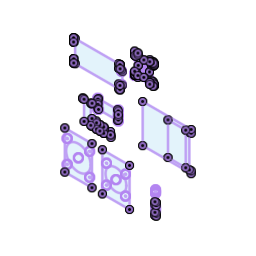
panels (Autodesk Fusion 360 design; units mm, degrees)
Autodesk Fusion 360 part; units mm, degrees
(part 1 of 2)
sketch "back construction" plane through (0, 0, 0) normal (0, 1, 0) x (1, 0, 0)
  line L0 (63.5, -61) -> (184.5, -61) construction
  line L1 (184.5, -61) -> (184.5, -120.5) construction
  line L2 (184.5, -120.5) -> (63.5, -120.5) construction
  line L3 (63.5, -120.5) -> (63.5, -61) construction
  line L4 (31.5, -5) -> (140.5, -5) construction
  line L5 (140.5, -5) -> (140.5, 39.5) construction
  line L6 (140.5, 39.5) -> (31.5, 39.5) construction
  line L7 (31.5, 39.5) -> (31.5, -5) construction
  line L8 (28.5, 32) -> (-8.5, 32)
  line L9 (-8.5, 32) -> (-8.5, -74)
  line L10 (-8.5, -74) -> (28.5, -74)
  line L11 (28.5, -74) -> (28.5, 32)
  line L12 (-15.5, -74) -> (35.5, -74)
  line L13 (35.5, -74) -> (35.5, -77)
  line L14 (35.5, -77) -> (-15.5, -77)
  line L15 (-15.5, -77) -> (-15.5, -74)
  line L16 (35, 34.5) -> (59, 34.5)
  line L17 (59, 34.5) -> (59, -3.5)
  line L18 (59, -3.5) -> (35, -3.5)
  line L19 (35, -3.5) -> (35, 34.5)
  line L20 (60.5, 34.5) -> (78.5, 34.5)
  line L21 (78.5, 34.5) -> (78.5, 4.5)
  line L22 (78.5, 4.5) -> (60.5, 4.5)
  line L23 (60.5, 4.5) -> (60.5, 34.5)
  line L24 (100, 34.5) -> (100, 4.5)
  line L25 (100, 4.5) -> (82, 4.5)
  line L26 (82, 4.5) -> (82, 34.5)
  line L27 (82, 34.5) -> (100, 34.5)
  line L28 (102, 34.5) -> (140, 34.5)
  line L29 (140, 34.5) -> (140, 23.5)
  line L30 (140, 23.5) -> (102, 23.5)
  line L31 (102, 23.5) -> (102, 34.5)
  line L32 (104.5, 23.5) -> (137.5, 23.5)
  line L33 (137.5, 23.5) -> (137.5, 7.5)
  line L34 (137.5, 7.5) -> (104.5, 7.5)
  line L35 (104.5, 7.5) -> (104.5, 23.5)
  circle A0 centre (180.5, -116.5) radius 4 construction
  circle A1 centre (180.5, -91) radius 4 construction
  circle A2 centre (180.5, -65) radius 4 construction
  circle A3 centre (67.5, -116.5) radius 4 construction
  circle A4 centre (67.5, -91) radius 4 construction
  circle A5 centre (67.5, -65) radius 4 construction
  line L36 (180.5, -116.5) -> (67.5, -116.5) construction
  line L37 (67.5, -116.5) -> (67.5, -65) construction
  line L38 (67.5, -65) -> (180.5, -65) construction
  line L39 (180.5, -65) -> (180.5, -116.5) construction
  line L40 (180.5, -95) -> (180.5, -112.5)
  line L41 (176.5, -116.5) -> (71.5, -116.5)
  line L42 (67.5, -112.5) -> (67.5, -95)
  line L43 (67.5, -87) -> (67.5, -69)
  line L44 (71.5, -65) -> (176.5, -65)
  line L45 (180.5, -69) -> (180.5, -87)
  arc A6 (180.5, -69) -> (176.5, -65) centre (180.5, -65) ccw
  line L46 (180.5, -65) -> (180.5, -69) construction
  line L47 (180.5, -65) -> (176.5, -65) construction
  arc A7 (176.5, -116.5) -> (180.5, -112.5) centre (180.5, -116.5) ccw
  line L48 (180.5, -116.5) -> (176.5, -116.5) construction
  line L49 (180.5, -116.5) -> (180.5, -112.5) construction
  arc A8 (67.5, -112.5) -> (71.5, -116.5) centre (67.5, -116.5) ccw
  line L50 (67.5, -116.5) -> (67.5, -112.5) construction
  line L51 (67.5, -116.5) -> (71.5, -116.5) construction
  arc A9 (67.5, -87) -> (67.5, -95) centre (67.5, -91) ccw
  line L52 (67.5, -91) -> (67.5, -87) construction
  line L53 (67.5, -91) -> (67.5, -95) construction
  arc A10 (71.5, -65) -> (67.5, -69) centre (67.5, -65) ccw
  line L54 (67.5, -65) -> (71.5, -65) construction
  line L55 (67.5, -65) -> (67.5, -69) construction
  arc A11 (180.5, -95) -> (180.5, -87) centre (180.5, -91) ccw
  line L56 (180.5, -91) -> (180.5, -95) construction
  line L57 (180.5, -91) -> (180.5, -87) construction
  line L58 (240.5, -148.5) -> (-54.5, -148.5)
  line L59 (-54.5, -148.5) -> (-54.5, 62.5)
  line L60 (-54.5, 62.5) -> (240.5, 62.5)
  line L61 (240.5, 62.5) -> (240.5, -148.5)
  dimension "d10" = 121
  dimension "d11" = 59.5
  dimension "d12" = 109
  dimension "d13" = 44.5
  dimension "d14" = 37
  dimension "d15" = 106
  dimension "d16" = 51
  dimension "d17" = 3
  dimension "d18" = 3
  dimension "d19" = 7
  dimension "d20" = 35
  dimension "d21" = 56
  dimension "d22" = 7.5
  dimension "d23" = 106
  dimension "d24" = 24
  dimension "d25" = 38
  dimension "d26" = 18
  dimension "d27" = 30
  dimension "d28" = 18
  dimension "d29" = 30
  dimension "d30" = 38
  dimension "d31" = 11
  dimension "d32" = 33
  dimension "d33" = 16
  dimension "d34" = 1.5
  dimension "d35" = 3.5
  dimension "d36" = 2
  dimension "d37" = 27
  dimension "d38" = 2.5
  dimension "d39" = 3.5
  dimension "d41" = 0
  dimension "d42" = 5
  dimension "d43" = 5
  dimension "d44" = 5
  dimension "d45" = 8
  dimension "d46" = 8
  dimension "d47" = 8
  dimension "d48" = 25.5
  dimension "d49" = 8
  dimension "d50" = 8
  dimension "d51" = 8
  dimension "d52" = 25.5
  dimension "d53" = 270
  dimension "d54" = 270
  dimension "d55" = 270
  dimension "d56" = 180
  dimension "d57" = 270
  dimension "d58" = 180
  dimension "height" = 295
  dimension "width" = 211
  dimension "d63" = 23
  dimension "d65" = 100
  constraint horizontal L0
  constraint vertical L1
  constraint horizontal L2
  constraint vertical L3
  constraint horizontal L4
  constraint vertical L5
  constraint horizontal L6
  constraint vertical L7
  constraint horizontal L8
  constraint vertical L9
  constraint horizontal L10
  constraint vertical L11
  constraint horizontal L12
  constraint vertical L13
  constraint horizontal L14
  constraint vertical L15
  constraint horizontal L16
  constraint vertical L17
  constraint horizontal L18
  constraint vertical L19
  constraint horizontal L20
  constraint vertical L21
  constraint horizontal L22
  constraint vertical L23
  constraint horizontal L27
  constraint vertical L24
  constraint horizontal L25
  constraint vertical L26
  constraint horizontal L28
  constraint vertical L29
  constraint horizontal L30
  constraint vertical L31
  constraint horizontal L32
  constraint vertical L33
  constraint horizontal L34
  constraint vertical L35
  constraint tangent L1 A0
  constraint tangent L2 A0
  constraint tangent L1 A2
  constraint tangent L0 A2
  constraint tangent L1 A1
  constraint tangent L3 A4
  constraint tangent L2 A3
  constraint tangent L3 A3
  constraint tangent L3 A5
  constraint tangent L0 A5
  constraint horizontal L36
  constraint vertical L37
  constraint horizontal L38
  constraint vertical L39
  constraint coincident A5.centre L37.end
  constraint coincident A0.centre L36.start
  constraint coincident A1 L40.start
  constraint coincident L39 L40.start
  constraint coincident L39 L40.end
  constraint coincident A0 L40.end
  constraint coincident A0 L41.start
  constraint coincident L36 L41.start
  constraint coincident A3 L41.end
  constraint coincident L36 L41.end
  constraint coincident L37 L42.start
  constraint coincident A3 L42.start
  constraint coincident A4 L42.end
  constraint coincident L37 L42.end
  constraint coincident A4 L43.start
  constraint coincident L37 L43.start
  constraint coincident A5 L43.end
  constraint coincident L37 L43.end
  constraint coincident A5 L44.start
  constraint coincident L38 L44.start
  constraint coincident A2 L44.end
  constraint coincident L38 L44.end
  constraint coincident L39 L45.start
  constraint coincident A2 L45.start
  constraint coincident L39 L45.end
  constraint coincident A1 L45.end
  constraint coincident A2.centre L38.end
  constraint coincident A3.centre L36.end
  constraint coincident A4.centre A9.centre
  constraint coincident A1.centre A11.centre
  constraint horizontal L58
  constraint vertical L59
  constraint horizontal L60
  constraint vertical L61
  measures "d10" distance of L0.start L0.end
  measures "d11" distance of L0.start L2.end
  measures "d12" distance of L4.start L4.end
  measures "d13" distance of L4.start L6.end
  measures "d14" distance of L8.start L8.end
  measures "d15" distance of L8.start L10.end
  measures "d16" distance of L12.start L12.end
  measures "d17" distance of L12.start L14.end
  measures "d18" distance of L7 L11
  measures "d19" distance of L9 L15
  measures "d20" distance of L3 L11
  measures "d21" distance of L0 L4
  measures "d22" distance of L6 L8
  measures "d23" distance of L8 L12
  measures "d24" distance of L16.start L16.end
  measures "d25" distance of L16.start L18.end
  measures "d26" distance of L20.start L20.end
  measures "d27" distance of L20.start L22.end
  measures "d28" distance of L26.end L24.start
  measures "d29" distance of L25.end L26.end
  measures "d30" distance of L28.start L28.end
  measures "d31" distance of L28.start L30.end
  measures "d32" distance of L32.start L32.end
  measures "d33" distance of L32.start L34.end
  measures "d34" distance of L17 L23
  measures "d35" distance of L21 L26
  measures "d36" distance of L24 L31
  measures "d37" distance of L28 L34
  measures "d38" distance of L31 L35
  measures "d39" distance of L7 L19
  measures "d41" distance of L27 L28
  measures "d42" distance of L6 L28
  measures "d43" distance of L6 L16
  measures "d44" distance of L6 L20
  measures "d45" diameter of A0
  measures "d46" diameter of A1
  measures "d47" diameter of A2
  measures "d48" distance of A0.centre A1.centre
  measures "d49" diameter of A3
  measures "d50" diameter of A4
  measures "d51" diameter of A5
  measures "d52" distance of A3.centre A4.centre
  measures "d56" angle of L52 L53
  measures "d58" angle of L56 L57
  measures "height" distance of L58.start L58.end
  measures "width" distance of L58.start L60.end
  measures "d63" distance of L6 L60
  measures "d65" distance of L5 L61
sketch "top construction" plane through (0, 0, 0) normal (0, 1, 0) x (1, 0, 0)
  line L0 (276, -385) -> (-88, -385)
  line L1 (-88, -385) -> (-88, -174)
  line L2 (-88, -174) -> (276, -174)
  line L3 (276, -174) -> (276, -385)
  line L4 (182, -339.5) -> (-58, -339.5)
  line L5 (-58, -339.5) -> (-58, -219.5)
  line L6 (-58, -219.5) -> (182, -219.5)
  line L7 (182, -219.5) -> (182, -339.5)
  line L8 (182, -317) -> (198, -317)
  line L9 (203, -312) -> (203, -247)
  line L10 (198, -242) -> (182, -242)
  line L11 (182, -242) -> (182, -317)
  arc A0 (198, -317) -> (203, -312) centre (198, -312) ccw
  arc A1 (203, -247) -> (198, -242) centre (198, -247) ccw
  line L12 (-65.5, -339) -> (-66.5, -339)
  line L13 (-66.5, -339) -> (-66.5, -319)
  line L14 (-66.5, -319) -> (-65.5, -319)
  line L15 (-65.5, -319) -> (-65.5, -339)
  line L16 (-65.5, -219) -> (-66.5, -219)
  line L17 (-66.5, -219) -> (-66.5, -239)
  line L18 (-66.5, -239) -> (-65.5, -239)
  line L19 (-65.5, -239) -> (-65.5, -219)
  line L20 (189.5, -339) -> (189.5, -319)
  line L21 (189.5, -239) -> (190.5, -239)
  line L22 (190.5, -239) -> (190.5, -219)
  line L23 (190.5, -219) -> (189.5, -219)
  line L24 (189.5, -319) -> (190.5, -319)
  line L25 (189.5, -219) -> (189.5, -239)
  line L26 (190.5, -319) -> (190.5, -339)
  line L27 (190.5, -339) -> (189.5, -339)
  point P0 (203, -317)
  dimension "d68" = 364
  dimension "d69" = 211
  dimension "d70" = 240
  dimension "d71" = 120
  dimension "d72" = 45.5
  dimension "d73" = 30
  dimension "d74" = 21
  dimension "d75" = 75
  dimension "d76" = 22.5
  dimension "d77" = 5
  dimension "d139" = 1
  dimension "d140" = 20
  dimension "d141" = 7.5
  dimension "d142" = 1
  dimension "d143" = 20
  dimension "d144" = 7.5
  dimension "d145" = 1
  dimension "d146" = 20
  dimension "d147" = 1
  dimension "d148" = 20
  dimension "d149" = 7.5
  dimension "d150" = 7.5
  constraint horizontal L0
  constraint vertical L1
  constraint horizontal L2
  constraint vertical L3
  constraint horizontal L4
  constraint vertical L5
  constraint horizontal L6
  constraint vertical L7
  constraint horizontal L8
  constraint vertical L9
  constraint horizontal L10
  constraint vertical L11
  constraint coincident L7 L8.start
  constraint coincident P0 L8
  constraint coincident P0 L9
  constraint tangent L8 A0
  constraint tangent L9 A0
  constraint tangent L9 A1
  constraint tangent L10 A1
  constraint equal A0 A1
  constraint horizontal L12
  constraint vertical L13
  constraint horizontal L14
  constraint vertical L15
  constraint horizontal L16
  constraint vertical L17
  constraint horizontal L18
  constraint vertical L19
  constraint horizontal L27
  constraint vertical L20
  constraint horizontal L24
  constraint vertical L26
  constraint horizontal L23
  constraint vertical L25
  constraint horizontal L21
  constraint vertical L22
  measures "d68" distance of L0.start L0.end
  measures "d69" distance of L0.start L2.end
  measures "d70" distance of L4.start L4.end
  measures "d71" distance of L4.start L6.end
  measures "d72" distance of L0 L4
  measures "d73" distance of L1 L5
  measures "d74" distance of L8.start P0
  measures "d75" distance of L8.start L10.end
  measures "d76" distance of L4 L8
  measures "d77" radius of A0
  measures "d139" distance of L12.start L12.end
  measures "d140" distance of L12.start L14.end
  measures "d141" distance of L5 L15
  measures "d142" distance of L16.start L16.end
  measures "d143" distance of L16.start L18.end
  measures "d144" distance of L5 L19
  measures "d145" distance of L26.end L20.start
  measures "d146" distance of L26.end L24.end
  measures "d147" distance of L22.end L23.end
  measures "d148" distance of L21.end L22.end
  measures "d149" distance of L7 L20
  measures "d150" distance of L7 L25
sketch "fans construction" plane through (0, 0, 0) normal (0, 1, 0) x (1, 0, 0)
  line L0 (242.5, 117.025) -> (92.5, 117.025)
  line L1 (92.5, 117.025) -> (92.5, 328.025)
  line L2 (92.5, 328.025) -> (242.5, 328.025)
  line L3 (242.5, 328.025) -> (242.5, 117.025)
  line L4 (35, 116.525) -> (-115, 116.525)
  line L5 (-115, 116.525) -> (-115, 327.525)
  line L6 (-115, 327.525) -> (35, 327.525)
  line L7 (35, 327.525) -> (35, 116.525)
  circle A0 centre (167.5, 222.525) radius 57.5
  circle A1 centre (-40, 222.025) radius 67.5
  line L8 (220, 170.025) -> (115, 170.025) construction
  line L9 (115, 170.025) -> (115, 275.025) construction
  line L10 (115, 275.025) -> (220, 275.025) construction
  line L11 (220, 275.025) -> (220, 170.025) construction
  line L12 (220, 170.025) -> (167.5, 170.025) construction
  line L13 (167.5, 170.025) -> (167.5, 222.525) construction
  line L14 (167.5, 222.525) -> (220, 222.525) construction
  line L15 (220, 222.525) -> (220, 170.025) construction
  circle A2 centre (220, 170.025) radius 2
  circle A3 centre (115, 170.025) radius 2
  circle A4 centre (220, 275.025) radius 2
  circle A5 centre (115, 275.025) radius 2
  line L16 (22, 160.025) -> (-102, 160.025) construction
  line L17 (-102, 160.025) -> (-102, 284.025) construction
  line L18 (-102, 284.025) -> (22, 284.025) construction
  line L19 (22, 284.025) -> (22, 160.025) construction
  line L20 (22, 160.025) -> (-40, 160.025) construction
  line L21 (-40, 160.025) -> (-40, 222.025) construction
  line L22 (-40, 222.025) -> (22, 222.025) construction
  line L23 (22, 222.025) -> (22, 160.025) construction
  circle A6 centre (22, 160.025) radius 2
  circle A7 centre (-102, 160.025) radius 2
  circle A8 centre (-102, 284.025) radius 2
  circle A9 centre (22, 284.025) radius 2
  dimension "d78" = 150
  dimension "d79" = 211
  dimension "d80" = 150
  dimension "d81" = 211
  dimension "d82" = 115
  dimension "d83" = 135
  dimension "d84" = 105.5
  dimension "d85" = 105.5
  dimension "d86" = 75
  dimension "d87" = 75
  dimension "d88" = 105
  dimension "d89" = 105
  dimension "d90" = 52.5
  dimension "d91" = 52.5
  dimension "d92" = 4
  dimension "d93" = 4
  dimension "d94" = 4
  dimension "d95" = 4
  dimension "d96" = 124
  dimension "d97" = 124
  dimension "d98" = 62
  dimension "d99" = 62
  dimension "d100" = 4
  dimension "d101" = 4
  dimension "d102" = 4
  dimension "d103" = 4
  constraint horizontal L0
  constraint vertical L1
  constraint horizontal L2
  constraint vertical L3
  constraint horizontal L4
  constraint vertical L5
  constraint horizontal L6
  constraint vertical L7
  constraint horizontal L8
  constraint vertical L9
  constraint horizontal L10
  constraint vertical L11
  constraint horizontal L12
  constraint vertical L13
  constraint horizontal L14
  constraint vertical L15
  constraint coincident A0.centre L13.end
  constraint coincident L8.start L11.end
  constraint coincident L8.end L9.start
  constraint coincident L10.end L11.start
  constraint coincident L9.end L10.start
  constraint horizontal L16
  constraint vertical L17
  constraint horizontal L18
  constraint vertical L19
  constraint horizontal L20
  constraint vertical L21
  constraint horizontal L22
  constraint vertical L23
  constraint coincident A1.centre L21.end
  constraint coincident L16.start L19.end
  constraint coincident L16.end L17.start
  constraint coincident L17.end L18.start
  constraint coincident L18.end L19.start
  measures "d78" distance of L0.start L0.end
  measures "d79" distance of L0.start L2.end
  measures "d80" distance of L4.start L4.end
  measures "d81" distance of L4.start L6.end
  measures "d82" diameter of A0
  measures "d83" diameter of A1
  measures "d84" distance of L0 A0.centre
  measures "d85" distance of L4 A1.centre
  measures "d86" distance of L1 A0.centre
  measures "d87" distance of L5 A1.centre
  measures "d88" distance of L8.start L8.end
  measures "d89" distance of L8.start L10.end
  measures "d90" distance of L8.start L12.end
  measures "d91" distance of L8.start L14.end
  measures "d92" diameter of A2
  measures "d93" diameter of A3
  measures "d94" diameter of A4
  measures "d95" diameter of A5
  measures "d96" distance of L16.start L16.end
  measures "d97" distance of L16.start L18.end
  measures "d98" distance of L16.start L20.end
  measures "d99" distance of L16.start L22.end
  measures "d100" diameter of A6
  measures "d101" diameter of A7
  measures "d102" diameter of A8
  measures "d103" diameter of A9
sketch "front construction" plane through (0, 0, 0) normal (0, 1, 0) x (1, 0, 0)
  line L0 (407.2786, 119.8333) -> (365.2786, 119.8333)
  line L1 (365.2786, 119.8333) -> (365.2786, 330.8333)
  line L2 (365.2786, 330.8333) -> (407.2786, 330.8333)
  line L3 (407.2786, 330.8333) -> (407.2786, 119.8333)
  line L4 (401.2786, 156.8333) -> (371.2786, 156.8333)
  line L5 (371.2786, 156.8333) -> (371.2786, 181.8333)
  line L6 (371.2786, 181.8333) -> (401.2786, 181.8333)
  line L7 (401.2786, 181.8333) -> (401.2786, 156.8333)
  line L8 (393.7786, 218.8333) -> (378.7786, 218.8333)
  line L9 (378.7786, 218.8333) -> (378.7786, 293.8333)
  line L10 (378.7786, 293.8333) -> (393.7786, 293.8333)
  line L11 (393.7786, 293.8333) -> (393.7786, 218.8333)
  circle A0 centre (386.2786, 162.3693) radius 4.5
  circle A1 centre (386.283, 172.3693) radius 3.5
  circle A2 centre (386.2786, 178.3693) radius 2
  line L12 (389.7786, 220.8333) -> (382.7786, 220.8333)
  line L13 (382.7786, 220.8333) -> (382.7786, 235.3333)
  line L14 (382.7786, 235.3333) -> (389.7786, 235.3333)
  line L15 (389.7786, 235.3333) -> (389.7786, 220.8333)
  line L16 (389.7786, 271.3333) -> (382.7786, 271.3333)
  line L17 (382.7786, 271.3333) -> (382.7786, 285.8333)
  line L18 (382.7786, 285.8333) -> (389.7786, 285.8333)
  line L19 (389.7786, 285.8333) -> (389.7786, 271.3333)
  circle A3 centre (386.2786, 245.3333) radius 3
  circle A4 centre (386.2786, 261.3333) radius 3
  dimension "d104" = 42
  dimension "d105" = 211
  dimension "d106" = 30
  dimension "d107" = 25
  dimension "d108" = 15
  dimension "d109" = 75
  dimension "d110" = 9
  dimension "d111" = 7
  dimension "d112" = 4
  dimension "d113" = 10
  dimension "d114" = 6
  dimension "d116" = 15
  dimension "d117" = 7
  dimension "d118" = 14.5
  dimension "d119" = 7
  dimension "d120" = 14.5
  dimension "d121" = 6
  dimension "d122" = 6
  dimension "d123" = 16
  dimension "d124" = 10
  dimension "d126" = 36
  dimension "d127" = 7.5
  dimension "d128" = 4
  dimension "d129" = 4
  dimension "d130" = 13.5
  dimension "d131" = 6
  dimension "d132" = 2
  dimension "d134" = 37
  dimension "d136" = 10
  dimension "d137" = 15
  dimension "d138" = 37
  constraint horizontal L0
  constraint vertical L1
  constraint horizontal L2
  constraint vertical L3
  constraint horizontal L4
  constraint vertical L5
  constraint horizontal L6
  constraint vertical L7
  constraint horizontal L8
  constraint vertical L9
  constraint horizontal L10
  constraint vertical L11
  constraint horizontal L12
  constraint vertical L13
  constraint horizontal L14
  constraint vertical L15
  constraint horizontal L16
  constraint vertical L17
  constraint horizontal L18
  constraint vertical L19
  measures "d104" distance of L0.start L0.end
  measures "d105" distance of L0.start L2.end
  measures "d106" distance of L4.start L4.end
  measures "d107" distance of L4.start L6.end
  measures "d108" distance of L8.start L8.end
  measures "d109" distance of L8.start L10.end
  measures "d110" diameter of A0
  measures "d111" diameter of A1
  measures "d112" diameter of A2
  measures "d113" distance of A0.centre A1.centre
  measures "d114" distance of A1.centre A2.centre
  measures "d116" distance of L7 A0.centre
  measures "d117" distance of L12.start L12.end
  measures "d118" distance of L12.start L14.end
  measures "d119" distance of L16.start L16.end
  measures "d120" distance of L16.start L18.end
  measures "d121" diameter of A3
  measures "d122" diameter of A4
  measures "d123" distance of A3.centre A4.centre
  measures "d124" distance of L14 A3.centre
  measures "d126" distance of L14 L16
  measures "d127" distance of L11 A3.centre
  measures "d128" distance of L11 L19
  measures "d129" distance of L11 L15
  measures "d130" distance of L1 L9
  measures "d131" distance of L1 L5
  measures "d132" distance of L8 L12
  measures "d134" distance of L2 L10
  measures "d136" distance of L16 A4.centre
  measures "d137" distance of L7 A2.centre
  measures "d138" distance of L0 L4
sketch "Skizze14" plane through (0, 0, 0) normal (0, 1, 0) x (1, 0, 0)
  circle A0 centre (330, 160) radius 4
  circle A1 centre (320, 160) radius 3
  dimension "d151" = 8
  dimension "d152" = 6
  measures "d151" diameter of A0
  measures "d152" diameter of A1
sketch "Skizze18" plane through (0, 0, 0) normal (0, 1, 0) x (1, 0, 0)
  line L0 (315, -225) -> (583, -225)
  line L1 (583, -225) -> (583, -14)
  line L2 (583, -14) -> (315, -14)
  line L3 (315, -14) -> (315, -225)
  line L4 (583, -207) -> (455, -207)
  line L5 (455, -207) -> (455, -27)
  line L6 (455, -27) -> (583, -27)
  line L7 (583, -27) -> (583, -207)
  line L8 (572.928, -207) -> (552.928, -207)
  line L9 (552.928, -207) -> (552.928, -27)
  line L10 (552.928, -27) -> (572.928, -27)
  line L11 (572.928, -27) -> (572.928, -207)
  dimension "d159" = 268
  dimension "d160" = 211
  dimension "d161" = 128
  dimension "d162" = 18
  dimension "d163" = 13
  dimension "d164" = 20
  constraint horizontal L0
  constraint vertical L1
  constraint horizontal L2
  constraint vertical L3
  constraint horizontal L4
  constraint vertical L5
  constraint horizontal L6
  constraint vertical L7
  constraint coincident L1 L4.start
  constraint horizontal L8
  constraint vertical L9
  constraint horizontal L10
  constraint vertical L11
  constraint coincident L4 L8.start
  measures "d159" distance of L0.start L0.end
  measures "d160" distance of L0.start L2.end
  measures "d161" distance of L4.start L4.end
  measures "d162" distance of L0 L4
  measures "d163" distance of L2 L6
  measures "d164" distance of L8.start L8.end
sketch "Skizze21" plane through (0, 0, 0) normal (0, 1, 0) x (1, 0, 0)
  line L0 (300.5747, -410.375) -> (342.5747, -410.375) construction
  line L1 (342.5747, -410.375) -> (342.5747, -360.375) construction
  line L2 (342.5747, -360.375) -> (300.5747, -360.375) construction
  line L3 (300.5747, -360.375) -> (300.5747, -410.375) construction
  circle A0 centre (300.5747, -410.375) radius 1.05
  circle A1 centre (342.5747, -410.375) radius 1.05
  circle A2 centre (342.5747, -360.375) radius 1.05
  circle A3 centre (300.5747, -360.375) radius 1.05
  circle A4 centre (290.8247, -423.625) radius 1.05
  circle A5 centre (352.3247, -347.125) radius 1.05
  line L4 (290.8247, -423.625) -> (352.3247, -423.625) construction
  circle A6 centre (290.8247, -347.125) radius 1.05
  line L5 (352.3247, -423.625) -> (352.3247, -347.125) construction
  line L6 (352.3247, -347.125) -> (290.8247, -347.125) construction
  circle A7 centre (352.3247, -423.625) radius 1.05
  line L7 (290.8247, -347.125) -> (290.8247, -423.625) construction
  line L8 (270.8247, -443.625) -> (372.375, -443.625)
  line L9 (372.375, -443.625) -> (372.375, -327.125)
  line L10 (372.375, -327.125) -> (270.8247, -327.125)
  line L11 (270.8247, -327.125) -> (270.8247, -443.625)
  line L12 (321.5747, -443.625) -> (321.5747, -327.125) construction
  line L13 (270.8247, -423.1299) -> (277.6357, -423.1301)
  line L14 (277.6357, -423.1301) -> (290.3673, -385.3833)
  line L15 (290.3673, -385.3833) -> (277.6305, -347.6245)
  line L16 (277.6305, -347.6245) -> (270.8247, -347.6245)
  line L17 (365.5137, -423.1301) -> (352.7821, -385.3833)
  line L18 (372.4852, -423.1301) -> (365.5137, -423.1301)
  line L19 (352.7821, -385.3833) -> (365.5189, -347.6245)
  line L20 (365.5189, -347.6245) -> (372.375, -347.6245)
  line L21 (274.8247, -430.3874) -> (270.8247, -432.6968)
  line L22 (270.8247, -432.6968) -> (270.8247, -437.3156)
  line L23 (270.8247, -437.3156) -> (274.8247, -439.625)
  line L24 (274.8247, -439.625) -> (278.8247, -437.3156)
  line L25 (278.8247, -437.3156) -> (278.8247, -432.6968)
  line L26 (278.8247, -432.6968) -> (274.8247, -430.3874)
  line L27 (270.8247, -385.375) -> (372.375, -385.375) construction
  line L28 (288.875, -434.666) -> (288.875, -441.125)
  line L29 (354.375, -443.625) -> (354.375, -434.666)
  line L30 (321.625, -427.088) -> (288.875, -434.666)
  line L31 (354.375, -434.666) -> (321.625, -427.088)
  line L32 (354.375, -441.125) -> (354.375, -434.666)
  line L33 (354.375, -434.666) -> (321.625, -427.088)
  line L34 (321.625, -427.088) -> (288.875, -434.666)
  line L35 (288.875, -434.666) -> (288.875, -443.625)
  line L36 (288.875, -336.084) -> (288.875, -327.125)
  line L37 (354.375, -336.084) -> (321.625, -343.6621)
  line L38 (321.625, -343.6621) -> (288.875, -336.084)
  line L39 (354.375, -329.625) -> (354.375, -336.084)
  line L40 (354.375, -327.125) -> (354.375, -336.084)
  line L41 (354.375, -336.084) -> (321.625, -343.6621)
  line L42 (321.625, -343.6621) -> (288.875, -336.084)
  line L43 (288.875, -336.084) -> (288.875, -329.625)
  line L44 (270.8247, -333.4429) -> (270.8345, -338.0617)
  line L45 (274.8198, -331.125) -> (270.8247, -333.4429)
  line L46 (278.8345, -338.0447) -> (278.8247, -333.4259)
  line L47 (270.8345, -338.0617) -> (274.8394, -340.3626)
  line L48 (278.8247, -333.4259) -> (274.8198, -331.125)
  line L49 (274.8394, -340.3626) -> (278.8345, -338.0447)
  line L50 (380.375, -437.3156) -> (380.375, -432.6968)
  line L51 (372.375, -432.6968) -> (372.375, -437.3156)
  line L52 (372.375, -437.3156) -> (376.375, -439.625)
  line L53 (376.375, -430.3874) -> (372.375, -432.6968)
  line L54 (380.375, -432.6968) -> (376.375, -430.3874)
  line L55 (376.375, -439.625) -> (380.375, -437.3156)
  line L56 (380.3651, -333.4259) -> (376.3602, -331.125)
  line L57 (376.3602, -331.125) -> (372.3652, -333.4429)
  line L58 (380.375, -338.0447) -> (380.3651, -333.4259)
  line L59 (372.3652, -333.4429) -> (372.375, -338.0617)
  line L60 (376.3799, -340.3626) -> (380.375, -338.0447)
  line L61 (372.375, -338.0617) -> (376.3799, -340.3626)
  point P0 (263.6908, -386.5389)
  point P1 (274.8247, -435.0062)
  point P2 (274.8637, -432.5062)
  point P3 (321.625, -441.625)
  point P4 (322.5681, -448.154)
  point P5 (321.625, -441.125)
  point P6 (321.625, -441.625)
  point P7 (321.5747, -327.125)
  point P8 (321.625, -329.625)
  point P9 (321.625, -329.125)
  point P10 (321.625, -329.125)
  point P11 (274.8296, -335.7438)
  point P12 (274.8637, -334.5062)
  point P13 (376.375, -435.0062)
  point P14 (376.8637, -432.5062)
  point P15 (376.3701, -335.7438)
  point P16 (376.8637, -334.5062)
  dimension "d198" = 42
  dimension "d199" = 50
  dimension "d200" = 2.1
  dimension "d201" = 2.1
  dimension "d202" = 2.1
  dimension "d203" = 2.1
  dimension "d204" = 61.5
  dimension "d205" = 76.5
  dimension "standoff_diam" = 2.1
  dimension "d207" = 2.1
  dimension "d208" = 2.1
  dimension "d209" = 2.1
  dimension "d210" = 9.75
  dimension "d211" = 13.25
  dimension "d212" = 20
  dimension "d213" = 20
  dimension "d215" = 20
  dimension "d220" = 21
  dimension "d221" = 4
  dimension "d222" = 4
  dimension "d223" = 25
  dimension "d231" = 4
  dimension "d232" = 4
  dimension "d233" = 4
  dimension "d234" = 4
  constraint horizontal L0
  constraint vertical L1
  constraint horizontal L2
  constraint vertical L3
  constraint coincident L0.start L3.end
  constraint coincident L0.end L1.start
  constraint coincident L1.end L2.start
  constraint coincident L2.end L3.start
  constraint horizontal L4
  constraint vertical L5
  constraint horizontal L6
  constraint vertical L7
  constraint coincident A4.centre L4.start
  constraint coincident L4.end L5.start
  constraint coincident A5.centre L5.end
  constraint coincident A6.centre L6.end
  constraint horizontal L8
  constraint vertical L9
  constraint horizontal L10
  constraint vertical L11
  constraint coincident L8 L12.start
  constraint coincident L10 P7
  constraint perpendicular L10 L12
  constraint symmetric L12 L13.end L17.start
  constraint symmetric L12 L15.end L19.end
  constraint symmetric L12 L14.end L17.end
  constraint parallel L11 L25
  constraint coincident L11 L27.start
  constraint coincident L9 L27.end
  constraint perpendicular L9 L27
  constraint symmetric L12.start L27 P7
  constraint symmetric L27 P6 P10
  constraint symmetric L27 L30.start L37.end
  constraint symmetric L27 L28.end L43.end
  constraint symmetric L27 L28.start L36.start
  constraint symmetric L27 L29.end L37.start
  constraint symmetric L27 L29.start L40.start
  constraint symmetric L27 L32.start L39.start
  constraint symmetric L27 P5 P8
  constraint symmetric L27 L35.end L36.end
  constraint coincident L17.start L18.end
  constraint coincident L9 L51.end
  constraint coincident L9 L59.end
  constraint coincident L11 L22.end
  constraint coincident L11 L44.start
  constraint coincident L10 L36.end
  constraint coincident L10 L40.start
  constraint coincident L11 L13.start
  constraint coincident L11 L16.end
  measures "d198" distance of L0.start L0.end
  measures "d199" distance of L0.start L2.end
  measures "d200" diameter of A0
  measures "d201" diameter of A1
  measures "d202" diameter of A2
  measures "d203" diameter of A3
  measures "d204" distance of L4.end A4.centre
  measures "d205" distance of A6.centre A4.centre
  measures "standoff_diam" diameter of A4
  measures "d207" diameter of A7
  measures "d208" diameter of A5
  measures "d209" diameter of A6
  measures "d210" distance of L3 L7
  measures "d211" distance of L0 L4
  measures "d212" distance of L4 L8
  measures "d213" distance of L7 L11
  measures "d215" distance of L6 L10
  measures "d220" distance of L3 L12
  measures "d221" distance of P1 L26
  measures "d222" distance of L8 L23.end
  measures "d223" distance of L0 L27
  measures "d231" distance of P11 L48
  measures "d232" distance of L10 L45.start
  measures "d233" distance of P13 L54
  measures "d234" distance of P15 L56
extrude "Extrude2" add sketch "front construction" sketch "top construction" sketch "fans construction" sketch "Skizze18" sketch "back construction" sketch "Skizze21" along normal blind 5 contours A0 | A1 | A2 | L12 L13 L14 L15 | L16 L17 L18 L19 | A3 | A4 of sketch 2 contours L4 L5 L6 L7 L11 | L7 L8 L9 L10 L11 A0 A1 | L12 L13 L14 L15 | L16 L17 L18 L19 | L20 L24 L26 L27 | L21 L22 L23 L25 of sketch 3 of sketch 4 contours L0 L1 L2 L3 L4 L5 L6 L8 L10 | L4 L6 L8 L9 L10 L11 of sketch 5 contours L8 L9 L10 L11 L12 | L10 L12 L13 L14 L15 | L16 L17 L18 L19 | L20 L21 L22 L23 | L24 L25 L26 L27 | L28 L29 L30 L31 L32 | L30 L32 L33 L34 L35 | L40 L41 L42 L43 L44 L45 A6 A7 A8 A9 A10 A11 of sketch 6 contours L8 L9 L10 L11 L13 L14 L15 L16 L17 L18 L19 L20 L21 L23 L24 L25 L26 L28 L29 L30 L31 L32 L33 L34 L35 L36 L37 L38 L39 L40 L41 L42 L43 L51 L57 L59 | L9 L50 L51 L52 L53 L54 L55 | L9 L57 L59 | L9 L56 L57 L58 L60 L61 makes body 1 at (141.5, 0, 79.6667) makes body 2 at (22, 0, 267) makes body 3 at (168.9323, 0, -133.0786) makes body 4 at (-41.6814, 0, -314.7954) makes body 5 at (387.4453, 0, -276.1667) makes body 6 at (115.5, 0, -12.8333) makes body 7 at (3.8333, 0, 3.3333) makes body 8 at (43, 0, -21.8333) makes body 9 at (88, 0, -14.5) makes body 10 at (72.5, 0, -14.5) makes body 11 at (-66.5, 1.6667, 332.3333) makes body 12 at (-65.5, 1.6667, 232.3333) makes body 13 at (189.5, 1.6667, 332.3333) makes body 14 at (189.5, 1.6667, 225.6667) makes body 15 at (361.6667, 0, 148.6667) makes body 16 at (382.05, 3.3333, -160.8302) makes body 17 at (387.4453, 0, -225.6667) makes body 18 at (387.6472, 3.3333, -248.003) makes body 19 at (387.231, 3.3333, -175.7385) makes body 20 at (384.3404, 3.3333, -178.8628) makes body 21 at (384.91, 3.3333, -264.003) makes body 22 at (314.7929, 0, 377.3208)
sketch "back projection" plane through (0, 0, 0) normal (0, 1, 0) x (1, 0, 0)
  line L0 (176.5, -116.5) -> (71.5, -116.5)
  arc A0 (67.5, -112.5) -> (71.5, -116.5) centre (67.5, -116.5) ccw
  line L1 (67.5, -112.5) -> (67.5, -95)
  arc A1 (67.5, -87) -> (67.5, -95) centre (67.5, -91) ccw
  line L2 (67.5, -87) -> (67.5, -69)
  arc A2 (71.5, -65) -> (67.5, -69) centre (67.5, -65) ccw
  line L3 (71.5, -65) -> (176.5, -65)
  arc A3 (180.5, -69) -> (176.5, -65) centre (180.5, -65) ccw
  line L4 (180.5, -69) -> (180.5, -87)
  arc A4 (180.5, -95) -> (180.5, -87) centre (180.5, -91) ccw
  line L5 (180.5, -95) -> (180.5, -112.5)
  arc A5 (176.5, -116.5) -> (180.5, -112.5) centre (180.5, -116.5) ccw
  line L6 (28.5, -74) -> (35.5, -74)
  line L7 (35.5, -74) -> (35.5, -77)
  line L8 (35.5, -77) -> (-15.5, -77)
  line L9 (-15.5, -77) -> (-15.5, -74)
  line L10 (-15.5, -74) -> (-8.5, -74)
  line L11 (-8.5, 32) -> (-8.5, -74)
  line L12 (28.5, 32) -> (-8.5, 32)
  line L13 (28.5, -74) -> (28.5, 32)
  line L14 (35, -3.5) -> (35, 34.5)
  line L15 (35, 34.5) -> (59, 34.5)
  line L16 (59, 34.5) -> (59, -3.5)
  line L17 (59, -3.5) -> (35, -3.5)
  line L18 (60.5, 4.5) -> (60.5, 34.5)
  line L19 (60.5, 34.5) -> (78.5, 34.5)
  line L20 (78.5, 34.5) -> (78.5, 4.5)
  line L21 (78.5, 4.5) -> (60.5, 4.5)
  line L22 (82, 34.5) -> (100, 34.5)
  line L23 (100, 34.5) -> (100, 4.5)
  line L24 (100, 4.5) -> (82, 4.5)
  line L25 (82, 4.5) -> (82, 34.5)
  line L26 (104.5, 7.5) -> (104.5, 23.5)
  line L27 (104.5, 23.5) -> (102, 23.5)
  line L28 (102, 23.5) -> (102, 34.5)
  line L29 (102, 34.5) -> (140, 34.5)
  line L30 (140, 34.5) -> (140, 23.5)
  line L31 (140, 23.5) -> (137.5, 23.5)
  line L32 (137.5, 23.5) -> (137.5, 7.5)
  line L33 (137.5, 7.5) -> (104.5, 7.5)
sketch "top projection" plane through (0, 0, 0) normal (0, 1, 0) x (1, 0, 0)
  line L0 (182, -317) -> (182, -339.5)
  line L1 (182, -339.5) -> (-58, -339.5)
  line L2 (-58, -339.5) -> (-58, -219.5)
  line L3 (-58, -219.5) -> (182, -219.5)
  line L4 (182, -219.5) -> (182, -242)
  line L5 (198, -242) -> (182, -242)
  arc A0 (203, -247) -> (198, -242) centre (198, -247) ccw
  line L6 (203, -312) -> (203, -247)
  arc A1 (198, -317) -> (203, -312) centre (198, -312) ccw
  line L7 (182, -317) -> (198, -317)
  line L8 (190.5, -339) -> (189.5, -339)
  line L9 (189.5, -339) -> (189.5, -319)
  line L10 (189.5, -319) -> (190.5, -319)
  line L11 (190.5, -319) -> (190.5, -339)
  line L12 (190.5, -219) -> (189.5, -219)
  line L13 (190.5, -239) -> (190.5, -219)
  line L14 (189.5, -239) -> (190.5, -239)
  line L15 (189.5, -219) -> (189.5, -239)
  line L16 (-66.5, -239) -> (-65.5, -239)
  line L17 (-66.5, -219) -> (-66.5, -239)
  line L18 (-65.5, -219) -> (-66.5, -219)
  line L19 (-65.5, -239) -> (-65.5, -219)
  line L20 (-65.5, -319) -> (-65.5, -339)
  line L21 (-65.5, -339) -> (-66.5, -339)
  line L22 (-66.5, -339) -> (-66.5, -319)
  line L23 (-66.5, -319) -> (-65.5, -319)
sketch "Skizze13" plane through (0, 0, 0) normal (0, 1, 0) x (1, 0, 0)
  line L0 (190.5, -339) -> (189.5, -339)
  line L1 (189.5, -339) -> (189.5, -319)
  line L2 (189.5, -319) -> (190.5, -319)
  line L3 (190.5, -319) -> (190.5, -339)
  line L4 (190.5, -219) -> (189.5, -219)
  line L5 (190.5, -239) -> (190.5, -219)
  line L6 (189.5, -239) -> (190.5, -239)
  line L7 (189.5, -219) -> (189.5, -239)
  line L8 (-66.5, -239) -> (-65.5, -239)
  line L9 (-66.5, -219) -> (-66.5, -239)
  line L10 (-65.5, -219) -> (-66.5, -219)
  line L11 (-65.5, -239) -> (-65.5, -219)
  line L12 (-65.5, -319) -> (-65.5, -339)
  line L13 (-65.5, -339) -> (-66.5, -339)
  line L14 (-66.5, -339) -> (-66.5, -319)
  line L15 (-66.5, -319) -> (-65.5, -319)
sketch "fan0 projection" plane through (0, 0, 0) normal (0, 1, 0) x (1, 0, 0)
  circle A0 centre (22, 160.025) radius 2
  circle A1 centre (22, 284.025) radius 2
  circle A2 centre (-102, 160.025) radius 2
  circle A3 centre (-40, 222.025) radius 67.5
  circle A4 centre (-102, 284.025) radius 2
  line L0 (35, 327.525) -> (35, 116.525)
  line L1 (35, 116.525) -> (-115, 116.525)
  line L2 (-115, 116.525) -> (-115, 327.525)
  line L3 (-115, 327.525) -> (35, 327.525)
sketch "fan1 projection" plane through (0, 0, 0) normal (0, 1, 0) x (1, 0, 0)
  circle A0 centre (115, 170.025) radius 2
  circle A1 centre (167.5, 222.525) radius 57.5
  circle A2 centre (220, 170.025) radius 2
  circle A3 centre (115, 275.025) radius 2
  circle A4 centre (220, 275.025) radius 2
  line L0 (242.5, 328.025) -> (242.5, 117.025)
  line L1 (242.5, 117.025) -> (92.5, 117.025)
  line L2 (92.5, 117.025) -> (92.5, 328.025)
  line L3 (92.5, 328.025) -> (242.5, 328.025)
sketch "Skizze15" plane through (0, 0, 0) normal (0, 1, 0) x (1, 0, 0)
  line L0 (382.7786, 285.8333) -> (389.7786, 285.8333)
  line L1 (389.7786, 285.8333) -> (389.7786, 271.3333)
  line L2 (389.7786, 271.3333) -> (382.7786, 271.3333)
  line L3 (382.7786, 271.3333) -> (382.7786, 285.8333)
  line L4 (382.7786, 235.3333) -> (389.7786, 235.3333)
  line L5 (389.7786, 235.3333) -> (389.7786, 220.8333)
  line L6 (389.7786, 220.8333) -> (382.7786, 220.8333)
  line L7 (382.7786, 220.8333) -> (382.7786, 235.3333)
  circle A0 centre (386.2786, 162.3693) radius 4.5
  circle A1 centre (386.283, 172.3693) radius 3.5
  circle A2 centre (386.2786, 178.3693) radius 2
  line L8 (382.7786, 235.3333) -> (389.7786, 235.3333)
  line L9 (389.7786, 235.3333) -> (389.7786, 220.8333)
  line L10 (389.7786, 220.8333) -> (382.7786, 220.8333)
  line L11 (382.7786, 220.8333) -> (382.7786, 235.3333)
  circle A3 centre (386.2786, 245.3333) radius 3
  circle A4 centre (386.2786, 261.3333) radius 3
  line L12 (389.7786, 285.8333) -> (382.7786, 285.8333)
  line L13 (382.7786, 285.8333) -> (382.7786, 271.3333)
  line L14 (382.7786, 271.3333) -> (389.7786, 271.3333)
  line L15 (389.7786, 271.3333) -> (389.7786, 285.8333)
sketch "Skizze19" plane through (0, 0, 0) normal (0, 1, 0) x (1, 0, 0)
  line L0 (455, -27) -> (455, -207)
  line L1 (583, -14) -> (583, -27)
  line L2 (583, -27) -> (572.928, -27)
  line L3 (572.928, -207) -> (583, -207)
  line L4 (583, -207) -> (583, -225)
  line L5 (583, -225) -> (315, -225)
  line L6 (315, -225) -> (315, -14)
  line L7 (315, -14) -> (583, -14)
  line L8 (455, -207) -> (552.928, -207)
  line L9 (552.928, -207) -> (552.928, -27)
  line L10 (552.928, -27) -> (455, -27)
  line L11 (572.928, -27) -> (572.928, -207)